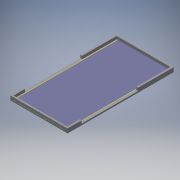
# Autodesk Inventor part: 30_Handyaufnahme
Saved by Autodesk Inventor 2016 (Build 200138000, 138)
## iProperties
Created: 2016-09-16
Part Number: 30_Handyaufnahme
Material: Generisch
Document SubType Name: Modeling
Designer: Bene
Density: 1 g/cm^3
Appearance: Vorgabe
Author: Bene
Autodesk Inventor part; units mm, degrees
(part 1 of 2)
ref_plane "YZ Plane" through (0, 0, 0) normal (1, 0, 0) x (0, 1, 0)
ref_plane "XZ Plane" through (0, 0, 0) normal (0, 1, 0) x (-1, 0, 0)
ref_plane "XY Plane" through (0, 0, 0) normal (0, 0, 1) x (1, 0, 0)
ref_plane "Arbeitsebene1" through (0, 0, 0) normal (0, 0, 1) x (1, 0, 0)
sketch "Skizze1" plane through (0, 0, 0) normal (0, 0, 1) x (1, 0, 0)
  line L0 (0, -3) -> (42, -3) projected
  line L1 (0, -61) -> (0, -3) projected
  line L2 (42, -61) -> (0, -61) projected
  line L3 (42, -3) -> (42, -61) projected
  point P0 (0, 0)
ref_plane "Arbeitsebene2" through (43.5, -39.6821, 19.9558) normal (0, 0, -1) x (-1, 0, 0)
sketch "Skizze2" plane through (43.5, -39.6821, 19.9558) normal (0, 0, -1) x (-1, 0, 0)
  spline S0 degree 3 poles (33.0112, -67.16) (33.0231, -67.1461) (33.0345, -67.1317) (33.045, -67.1168) knots 0 0 0 0 1 1 1 1 construction
  line L0 (33.045, -67.1168) -> (33.045, 67.1168) construction
  spline S1 degree 3 poles (33.045, 67.1168) (33.0378, 67.127) (33.0303, 67.1369) (33.0224, 67.1465) (33.0188, 67.1511) (33.015, 67.1555) (33.0113, 67.16) knots 0 0 0 0 0.680527 0.680527 0.680527 1 1 1 1 construction
  line L1 (33.0113, 67.16) -> (-33.0112, 67.16) construction
  spline S2 degree 3 poles (-33.0112, 67.16) (-33.0231, 67.1461) (-33.0345, 67.1317) (-33.045, 67.1168) knots 0 0 0 0 1 1 1 1 construction
  line L2 (-33.045, 67.1168) -> (-33.045, -67.1168) construction
  spline S3 degree 3 poles (-33.045, -67.1168) (-33.0378, -67.127) (-33.0303, -67.1369) (-33.0224, -67.1465) (-33.0188, -67.1511) (-33.015, -67.1555) (-33.0113, -67.16) knots 0 0 0 0 0.680527 0.680527 0.680527 1 1 1 1 construction
  line L3 (-33.0113, -67.16) -> (33.0112, -67.16) construction
  circle A0 centre (20, -51.9963) radius 1.9005 construction
  circle A1 centre (20, -59.8179) radius 3.8131 construction
  line L4 (-6.8399, -3.5028) -> (-6.8399, -3.3752) construction
  line L5 (-8.0242, -3.5028) -> (-6.8399, -3.5028) construction
  line L6 (-8.0242, -3.3752) -> (-8.0242, -3.5028) construction
  line L7 (-7.8023, -3.3745) -> (-8.0242, -3.3752) construction
  spline S4 degree 3 poles (-7.4456, -3.2197) (-7.4554, -3.2338) (-7.4745, -3.2614) (-7.5108, -3.295) (-7.5488, -3.3237) (-7.5917, -3.3439) (-7.638, -3.3581) (-7.6886, -3.3688) (-7.7439, -3.374) (-7.7824, -3.3743) (-7.8023, -3.3745) knots 0 0 0 0 0.125872 0.246008 0.361529 0.474729 0.592378 0.717307 0.853877 1 1 1 1 construction
  line L8 (-6.2942, -1.4127) -> (-7.4456, -3.2197) construction
  line L9 (-6.2936, -0.4264) -> (-6.2942, -1.4127) construction
  spline S5 degree 3 poles (-6.5588, -0.1303) (-6.5345, -0.1322) (-6.4894, -0.1356) (-6.4278, -0.1541) (-6.3782, -0.1841) (-6.344, -0.2264) (-6.3204, -0.2731) (-6.3032, -0.3223) (-6.2942, -0.3738) (-6.2938, -0.4088) (-6.2936, -0.4264) knots 0 0 0 0 0.16126 0.299397 0.422694 0.539052 0.654895 0.768299 0.88344 1 1 1 1 construction
  line L10 (-6.8508, -0.1303) -> (-6.5588, -0.1303) construction
  line L11 (-6.8508, -0.0028) -> (-6.8508, -0.1303) construction
  line L12 (-5.5009, -0.0028) -> (-6.8508, -0.0028) construction
  line L13 (-5.5009, -0.1303) -> (-5.5009, -0.0028) construction
  line L14 (-5.7867, -0.1303) -> (-5.5009, -0.1303) construction
  spline S6 degree 3 poles (-6.0406, -0.4267) (-6.0397, -0.405) (-6.0379, -0.3639) (-6.0275, -0.3052) (-6.007, -0.2542) (-5.98, -0.2099) (-5.9439, -0.1741) (-5.8986, -0.1488) (-5.8453, -0.1333) (-5.8069, -0.1314) (-5.7867, -0.1303) knots 0 0 0 0 0.146323 0.278524 0.401374 0.515931 0.627633 0.741117 0.863359 1 1 1 1 construction
  line L15 (-6.0406, -1.3884) -> (-6.0406, -0.4267) construction
  line L16 (-4.918, -3.161) -> (-6.0406, -1.3884) construction
  spline S7 degree 3 poles (-4.535, -3.3752) (-4.5587, -3.374) (-4.6039, -3.3717) (-4.6681, -3.362) (-4.7245, -3.344) (-4.7731, -3.3185) (-4.8158, -3.2871) (-4.8537, -3.2502) (-4.8882, -3.208) (-4.9079, -3.1769) (-4.918, -3.161) knots 0 0 0 0 0.153768 0.293392 0.419393 0.535968 0.647417 0.761826 0.877861 1 1 1 1 construction
  line L17 (-4.3245, -3.3752) -> (-4.535, -3.3752) construction
  line L18 (-4.3245, -3.5028) -> (-4.3245, -3.3752) construction
  line L19 (-5.6898, -3.5028) -> (-4.3245, -3.5028) construction
  line L20 (-5.6898, -3.3752) -> (-5.6898, -3.5028) construction
  line L21 (-5.3548, -3.3745) -> (-5.6898, -3.3752) construction
  spline S8 degree 3 poles (-5.1551, -3.2969) (-5.1567, -3.3057) (-5.1597, -3.3228) (-5.1771, -3.3435) (-5.2009, -3.3587) (-5.2422, -3.3674) (-5.2937, -3.3754) (-5.3353, -3.3748) (-5.3548, -3.3745) knots 0 0 0 0 0.113211 0.218392 0.333929 0.468642 0.751865 1 1 1 1 construction
  spline S9 degree 3 poles (-5.2257, -3.1614) (-5.2152, -3.1742) (-5.1958, -3.1977) (-5.1744, -3.2339) (-5.1598, -3.2663) (-5.1566, -3.2873) (-5.1551, -3.2969) knots 0 0 0 0 0.319442 0.590352 0.813067 1 1 1 1 construction
  line L22 (-6.2146, -1.5827) -> (-5.2257, -3.1614) construction
  line L23 (-7.2559, -3.2192) -> (-6.2146, -1.5827) construction
  spline S10 degree 3 poles (-7.283, -3.3017) (-7.2809, -3.2898) (-7.2757, -3.2611) (-7.2632, -3.2346) (-7.2559, -3.2192) knots 0 0 0 0 0.415019 1 1 1 1 construction
  spline S11 degree 3 poles (-7.1806, -3.3752) (-7.1943, -3.3741) (-7.219, -3.372) (-7.2524, -3.359) (-7.2756, -3.334) (-7.2804, -3.3128) (-7.283, -3.3017) knots 0 0 0 0 0.295689 0.535244 0.758161 1 1 1 1 construction
  line L24 (-6.8399, -3.3752) -> (-7.1806, -3.3752) construction
  spline S12 degree 3 poles (-3.5022, -3.1566) (-3.5031, -3.1731) (-3.5048, -3.205) (-3.519, -3.2499) (-3.5424, -3.2883) (-3.5742, -3.3199) (-3.6132, -3.344) (-3.6573, -3.3625) (-3.7074, -3.3727) (-3.7425, -3.3739) (-3.7608, -3.3745) knots 0 0 0 0 0.130398 0.250624 0.365732 0.481486 0.600063 0.724028 0.85602 1 1 1 1 construction
  line L25 (-3.5022, -0.0028) -> (-3.5022, -3.1566) construction
  line L26 (-3.3463, -0.0028) -> (-3.5022, -0.0028) construction
  line L27 (-3.0592, -0.4024) -> (-3.3463, -0.0028) construction
  line L28 (-0.9728, -3.2294) -> (-3.0592, -0.4024) construction
  line L29 (-0.9728, -0.441) -> (-0.9728, -3.2294) construction
  spline S13 degree 3 poles (-1.2708, -0.1303) (-1.2481, -0.1313) (-1.205, -0.1332) (-1.1444, -0.1496) (-1.0921, -0.1758) (-1.0489, -0.2131) (-1.014, -0.2586) (-0.9913, -0.3135) (-0.9749, -0.3746) (-0.9736, -0.4182) (-0.9728, -0.441) knots 0 0 0 0 0.139526 0.264775 0.383096 0.497107 0.612888 0.732612 0.860253 1 1 1 1 construction
  line L30 (-1.4768, -0.1303) -> (-1.2708, -0.1303) construction
  line L31 (-1.4768, -0.0028) -> (-1.4768, -0.1303) construction
  line L32 (-0.2882, -0.0028) -> (-1.4768, -0.0028) construction
  line L33 (-0.2882, -0.1303) -> (-0.2882, -0.0028) construction
  line L34 (-0.5201, -0.1303) -> (-0.2882, -0.1303) construction
  spline S14 degree 3 poles (-0.8009, -0.4412) (-0.7987, -0.4165) (-0.7944, -0.3696) (-0.7729, -0.3049) (-0.7416, -0.2496) (-0.6986, -0.2065) (-0.6522, -0.1738) (-0.6072, -0.1485) (-0.5631, -0.1336) (-0.5341, -0.1314) (-0.5201, -0.1303) knots 0 0 0 0 0.161786 0.306268 0.440748 0.572979 0.699363 0.810681 0.908913 1 1 1 1 construction
  line L35 (-0.8009, -3.1464) -> (-0.8009, -0.4412) construction
  spline S15 degree 3 poles (-0.5473, -3.3752) (-0.559, -3.375) (-0.5837, -3.3746) (-0.6221, -3.3685) (-0.6624, -3.3541) (-0.705, -3.337) (-0.7459, -3.3091) (-0.7757, -3.2652) (-0.795, -3.2098) (-0.7988, -3.1685) (-0.8009, -3.1464) knots 0 0 0 0 0.091352 0.191475 0.301121 0.422609 0.548749 0.678857 0.82774 1 1 1 1 construction
  line L36 (-0.2882, -3.3752) -> (-0.5473, -3.3752) construction
  line L37 (-0.2882, -3.5028) -> (-0.2882, -3.3752) construction
  line L38 (-1.0811, -3.5028) -> (-0.2882, -3.5028) construction
  line L39 (-3.3302, -0.4752) -> (-1.0811, -3.5028) construction
  line L40 (-3.3302, -3.1561) -> (-3.3302, -0.4752) construction
  spline S16 degree 3 poles (-3.0592, -3.3752) (-3.0768, -3.3747) (-3.1108, -3.3737) (-3.1602, -3.3656) (-3.2056, -3.3499) (-3.2475, -3.3292) (-3.2835, -3.2996) (-3.31, -3.2597) (-3.3257, -3.2106) (-3.3286, -3.1749) (-3.3302, -3.1561) knots 0 0 0 0 0.133425 0.258235 0.378828 0.497512 0.612266 0.728756 0.856573 1 1 1 1 construction
  line L41 (-2.8208, -3.3752) -> (-3.0592, -3.3752) construction
  line L42 (-2.8208, -3.5028) -> (-2.8208, -3.3752) construction
  line L43 (-4.0148, -3.5028) -> (-2.8208, -3.5028) construction
  line L44 (-4.0148, -3.3752) -> (-4.0148, -3.5028) construction
  line L45 (-3.7608, -3.3745) -> (-4.0148, -3.3752) construction
  line L46 (-7.4524, 47.564) -> (-6.685, 47.564) construction
  line L47 (-8.7169, 51.0791) -> (-7.4524, 47.564) construction
  line L48 (-8.0576, 51.0791) -> (-8.7169, 51.0791) construction
  line L49 (-7.6848, 50.0505) -> (-8.0576, 51.0791) construction
  line L50 (-6.4202, 50.0505) -> (-7.6848, 50.0505) construction
  line L51 (-6.0636, 51.0791) -> (-6.4202, 50.0505) construction
  line L52 (-5.4206, 51.0791) -> (-6.0636, 51.0791) construction
  line L53 (-6.685, 47.564) -> (-5.4206, 51.0791) construction
  line L54 (-4.2355, 51.0663) -> (-4.8651, 51.0663) construction
  line L55 (-4.2355, 47.5663) -> (-4.2355, 51.0663) construction
  line L56 (-4.8651, 47.5663) -> (-4.2355, 47.5663) construction
  line L57 (-4.8651, 51.0663) -> (-4.8651, 47.5663) construction
  line L58 (4.4914, 49.7461) -> (4.4911, 49.7461) construction
  line L59 (4.4911, 51.0604) -> (4.4911, 49.7461) construction
  line L60 (5.1173, 51.0604) -> (4.4911, 51.0604) construction
  line L61 (5.1177, 47.6325) -> (5.1173, 51.0604) construction
  spline S17 degree 3 poles (4.1058, 47.5637) (4.1579, 47.5645) (4.2591, 47.566) (4.4066, 47.5698) (4.5455, 47.5757) (4.676, 47.5838) (4.7984, 47.5928) (4.9124, 47.6039) (5.018, 47.6171) (5.0853, 47.6275) (5.1177, 47.6325) knots 0 0 0 0 0.153776 0.299112 0.436052 0.564635 0.685507 0.798759 0.903163 1 1 1 1 construction
  spline S18 degree 3 poles (2.9597, 47.8428) (2.9927, 47.8202) (3.0604, 47.7738) (3.1743, 47.7175) (3.2997, 47.6694) (3.4373, 47.6297) (3.5873, 47.5995) (3.7496, 47.5793) (3.9237, 47.5654) (4.0438, 47.5643) (4.1058, 47.5637) knots 0 0 0 0 0.100077 0.205184 0.316963 0.435866 0.563106 0.699421 0.844937 1 1 1 1 construction
  spline S19 degree 3 poles (2.5847, 48.5888) (2.5862, 48.55) (2.5893, 48.474) (2.6081, 48.3629) (2.6392, 48.258) (2.6824, 48.1595) (2.7369, 48.0683) (2.8007, 47.984) (2.8751, 47.908) (2.9313, 47.8647) (2.9597, 47.8428) knots 0 0 0 0 0.134405 0.262714 0.388354 0.511556 0.633904 0.754637 0.876442 1 1 1 1 construction
  spline S20 degree 3 poles (4.1382, 49.7125) (4.0897, 49.7125) (3.9939, 49.7125) (3.8519, 49.7012) (3.7137, 49.6833) (3.5795, 49.6557) (3.449, 49.6206) (3.3219, 49.578) (3.199, 49.5259) (3.0807, 49.4666) (2.9695, 49.3986) (2.8724, 49.3163) (2.7883, 49.2235) (2.7192, 49.1185) (2.664, 49.002) (2.6224, 48.8745) (2.5952, 48.7354) (2.5882, 48.6388) (2.5847, 48.5888) knots 0 0 0 0 0.067532 0.133398 0.198121 0.261385 0.324001 0.386218 0.447841 0.509748 0.570295 0.628891 0.686268 0.74407 0.803241 0.865264 0.930334 1 1 1 1 construction
  spline S21 degree 3 poles (4.2556, 49.7112) (4.2484, 49.7115) (4.2093, 49.7126) (4.1702, 49.7125) (4.1382, 49.7125) knots 0 0 0 0 0.18275 1 1 1 1 construction
  line L62 (4.2556, 49.7112) -> (4.2556, 49.3014) construction
  spline S22 degree 3 poles (4.1382, 49.3018) (4.1728, 49.3022) (4.212, 49.3026) (4.2511, 49.3016) (4.2556, 49.3014) knots 0 0 0 0 0.884897 1 1 1 1 construction
  spline S23 degree 3 poles (3.2143, 48.6113) (3.2153, 48.6385) (3.2172, 48.6913) (3.2291, 48.7679) (3.2493, 48.8395) (3.2762, 48.9065) (3.3108, 48.9685) (3.353, 49.0254) (3.4031, 49.0771) (3.4601, 49.1241) (3.5239, 49.1657) (3.5937, 49.2025) (3.67, 49.2324) (3.752, 49.2577) (3.84, 49.2775) (3.9342, 49.291) (4.0342, 49.2998) (4.1029, 49.3011) (4.1382, 49.3018) knots 0 0 0 0 0.06256 0.121668 0.178098 0.23345 0.287556 0.341282 0.39623 0.45286 0.511168 0.571359 0.634254 0.699626 0.76886 0.841752 0.918713 1 1 1 1 construction
  spline S24 degree 3 poles (4.0675, 47.9797) (4.0361, 47.9802) (3.9752, 47.9813) (3.8859, 47.9885) (3.8016, 48.0011) (3.7218, 48.0179) (3.6473, 48.0409) (3.577, 48.0674) (3.512, 48.1003) (3.4517, 48.137) (3.397, 48.1787) (3.3489, 48.2258) (3.3086, 48.2784) (3.2748, 48.3352) (3.2492, 48.3975) (3.2299, 48.4645) (3.218, 48.5364) (3.2156, 48.5859) (3.2143, 48.6113) knots 0 0 0 0 0.078508 0.152812 0.224327 0.292184 0.35687 0.41968 0.480233 0.539284 0.596432 0.652316 0.707476 0.761976 0.817709 0.875782 0.936291 1 1 1 1 construction
  spline S25 degree 3 poles (4.4911, 48.011) (4.4798, 48.0091) (4.4552, 48.0052) (4.4157, 47.9988) (4.3706, 47.9949) (4.3204, 47.9896) (4.2648, 47.9871) (4.2037, 47.9831) (4.1373, 47.9817) (4.0913, 47.9804) (4.0675, 47.9797) knots 0 0 0 0 0.081247 0.175609 0.281928 0.400632 0.531508 0.674808 0.831962 1 1 1 1 construction
  line L63 (4.4914, 49.2753) -> (4.4911, 48.011) construction
  line L64 (4.4914, 49.2753) -> (4.4914, 49.7461) construction
  line L65 (1.1321, 49.4618) -> (1.1321, 49.0439) construction
  line L66 (-0.1445, 49.0439) -> (1.1321, 49.0439) construction
  line L67 (-0.1445, 49.4618) -> (-0.1445, 49.0439) construction
  line L68 (1.1321, 49.4618) -> (-0.1445, 49.4618) construction
  line L69 (1.3148, 48.0227) -> (-0.2317, 48.0227) construction
  line L70 (1.3148, 50.6523) -> (1.3148, 48.0227) construction
  line L71 (-0.3242, 50.6523) -> (1.3148, 50.6523) construction
  line L72 (-0.3242, 51.0703) -> (-0.3242, 50.6523) construction
  line L73 (1.9444, 51.0703) -> (-0.3242, 51.0703) construction
  line L74 (1.9444, 47.6047) -> (1.9444, 51.0703) construction
  line L75 (-0.2317, 47.6047) -> (1.9444, 47.6047) construction
  line L76 (-0.2317, 48.0227) -> (-0.2317, 47.6047) construction
  line L77 (12.0011, -59.9793) -> (13.1916, -59.9793) construction
  line L78 (12.0016, -58.7456) -> (12.0011, -59.9793) construction
  spline S26 degree 3 poles (13.0636, -58.6238) (13.008, -58.6247) (12.8994, -58.6265) (12.7403, -58.6348) (12.5887, -58.6465) (12.4674, -58.6614) (12.3752, -58.6739) (12.3107, -58.684) (12.25, -58.6938) (12.193, -58.7037) (12.1398, -58.7141) (12.0903, -58.7244) (12.0446, -58.7348) (12.0156, -58.7421) (12.0016, -58.7456) knots 0 0 0 0 0.1557 0.304053 0.446066 0.581493 0.646038 0.70672 0.764353 0.818072 0.868837 0.916143 0.959573 1 1 1 1 construction
  spline S27 degree 3 poles (14.8994, -59.8671) (14.9015, -59.8386) (14.9058, -59.7804) (14.896, -59.691) (14.8756, -59.5986) (14.8423, -59.5034) (14.7975, -59.4054) (14.7407, -59.3045) (14.6723, -59.2006) (14.6072, -59.1128) (14.5468, -59.0432) (14.4936, -58.9936) (14.4336, -58.9473) (14.3673, -58.9037) (14.2943, -58.8638) (14.215, -58.8263) (14.1292, -58.7919) (14.0364, -58.7615) (13.9375, -58.7331) (13.8319, -58.7081) (13.7198, -58.6866) (13.6013, -58.6678) (13.4762, -58.6516) (13.3445, -58.639) (13.2062, -58.6296) (13.1118, -58.6257) (13.0636, -58.6238) knots 0 0 0 0 0.03432 0.070095 0.107736 0.147992 0.191058 0.237276 0.287084 0.340654 0.368703 0.397784 0.428021 0.459755 0.493076 0.528071 0.565217 0.604154 0.645525 0.688944 0.734677 0.782823 0.833245 0.886343 0.941974 1 1 1 1 construction
  spline S28 degree 3 poles (12.97, -61.1861) (13.0055, -61.1857) (13.0754, -61.1849) (13.1791, -61.1799) (13.2802, -61.173) (13.3788, -61.163) (13.4748, -61.1509) (13.5681, -61.1357) (13.6586, -61.1177) (13.7468, -61.0975) (13.8322, -61.0745) (13.915, -61.0482) (13.9954, -61.0202) (14.0729, -60.9887) (14.1481, -60.9554) (14.2206, -60.9189) (14.2904, -60.8797) (14.3574, -60.8382) (14.4214, -60.7945) (14.481, -60.7477) (14.5374, -60.6994) (14.5891, -60.6482) (14.6377, -60.5956) (14.6809, -60.5398) (14.7215, -60.4828) (14.7574, -60.4231) (14.789, -60.3611) (14.817, -60.2971) (14.8412, -60.2309) (14.861, -60.1623) (14.8765, -60.0916) (14.8882, -60.0187) (14.8966, -59.9437) (14.8984, -59.8928) (14.8994, -59.8671) knots 0 0 0 0 0.04072 0.080388 0.119206 0.157214 0.194247 0.23036 0.265776 0.30032 0.33425 0.367443 0.400064 0.432052 0.463561 0.494554 0.525258 0.555487 0.58515 0.614287 0.642511 0.670405 0.697816 0.724748 0.751504 0.77813 0.804755 0.831413 0.858375 0.88569 0.913305 0.941536 0.97047 1 1 1 1 construction
  spline S29 degree 3 poles (12.1025, -61.0811) (12.1275, -61.0888) (12.1807, -61.1053) (12.2668, -61.1251) (12.3633, -61.1429) (12.4695, -61.1584) (12.5844, -61.1704) (12.7068, -61.1792) (12.8361, -61.1851) (12.9247, -61.1858) (12.97, -61.1861) knots 0 0 0 0 0.089617 0.19034 0.302104 0.425118 0.55728 0.697152 0.844869 1 1 1 1 construction
  line L79 (12.2284, -60.7657) -> (12.1025, -61.0811) construction
  spline S30 degree 3 poles (12.97, -60.863) (12.9289, -60.8627) (12.85, -60.8621) (12.7364, -60.856) (12.6323, -60.8482) (12.5375, -60.8356) (12.4508, -60.8206) (12.3708, -60.805) (12.2972, -60.7866) (12.2507, -60.7725) (12.2284, -60.7657) knots 0 0 0 0 0.164208 0.315374 0.454233 0.581106 0.697247 0.80569 0.906846 1 1 1 1 construction
  spline S31 degree 3 poles (14.2999, -59.8832) (14.2981, -59.9225) (14.2946, -59.9992) (14.2748, -60.1101) (14.2447, -60.2138) (14.2029, -60.3098) (14.1501, -60.3984) (14.086, -60.4795) (14.011, -60.5531) (13.9249, -60.618) (13.8303, -60.6754) (13.7282, -60.7257) (13.6189, -60.768) (13.5027, -60.8031) (13.3794, -60.8298) (13.2492, -60.8489) (13.112, -60.8611) (13.0181, -60.8623) (12.97, -60.863) knots 0 0 0 0 0.063442 0.123831 0.181341 0.237349 0.292409 0.347434 0.403696 0.461553 0.521105 0.582039 0.645058 0.710115 0.777776 0.848453 0.922443 1 1 1 1 construction
  spline S32 degree 3 poles (13.0442, -58.9209) (13.0901, -58.9217) (13.1796, -58.9234) (13.3102, -58.9354) (13.434, -58.9546) (13.5509, -58.9814) (13.6609, -59.0158) (13.764, -59.0579) (13.8602, -59.1076) (13.9493, -59.1646) (14.0298, -59.2291) (14.1004, -59.3012) (14.1599, -59.381) (14.2094, -59.4675) (14.2484, -59.5615) (14.2764, -59.6626) (14.2948, -59.7706) (14.2982, -59.845) (14.2999, -59.8832) knots 0 0 0 0 0.077186 0.150659 0.220703 0.287908 0.352389 0.41457 0.475162 0.534436 0.592319 0.648565 0.703868 0.759442 0.816014 0.874682 0.935701 1 1 1 1 construction
  spline S33 degree 3 poles (12.5416, -58.9736) (12.5536, -58.9695) (12.5799, -58.9606) (12.624, -58.9513) (12.6754, -58.9429) (12.7343, -58.9352) (12.801, -58.9301) (12.8753, -58.925) (12.9573, -58.9226) (13.0144, -58.9215) (13.0442, -58.9209) knots 0 0 0 0 0.07529 0.164091 0.266069 0.383443 0.515244 0.661769 0.823927 1 1 1 1 construction
  line L80 (12.5416, -59.6822) -> (12.5416, -58.9736) construction
  line L81 (13.1916, -59.6822) -> (12.5416, -59.6822) construction
  line L82 (13.1916, -59.9793) -> (13.1916, -59.6822) construction
  line L83 (14.6059, -57.957) -> (14.5472, -58.0596) construction
  line L84 (14.5472, -58.0596) -> (14.3623, -58.0596) construction
  line L85 (14.3623, -58.0596) -> (14.3623, -57.0596) construction
  line L86 (14.3623, -57.0596) -> (14.4521, -57.0596) construction
  line L87 (14.4521, -57.0596) -> (14.4521, -57.957) construction
  line L88 (14.4521, -57.957) -> (14.6059, -57.957) construction
  spline S34 degree 3 poles (13.028, -57.9827) (13.0358, -57.9825) (13.0512, -57.9821) (13.0737, -57.9792) (13.0953, -57.9747) (13.1157, -57.9677) (13.1353, -57.9594) (13.1536, -57.9488) (13.1712, -57.9366) (13.1876, -57.9224) (13.2025, -57.9063) (13.2161, -57.8889) (13.2277, -57.8697) (13.2379, -57.8492) (13.2457, -57.8269) (13.2524, -57.8033) (13.2572, -57.7781) (13.2589, -57.7608) (13.2598, -57.7519) knots 0 0 0 0 0.064442 0.126553 0.186779 0.245944 0.30411 0.361785 0.420255 0.479943 0.540286 0.600712 0.661962 0.724472 0.788881 0.856306 0.926348 1 1 1 1 construction
  line L89 (13.2598, -57.7519) -> (13.3495, -57.7519) construction
  spline S35 degree 3 poles (13.3495, -57.7519) (13.3489, -57.7638) (13.3478, -57.7872) (13.3424, -57.8213) (13.3347, -57.8539) (13.3238, -57.8847) (13.3104, -57.9141) (13.2939, -57.9417) (13.2747, -57.9677) (13.2529, -57.9918) (13.2293, -58.0137) (13.204, -58.0329) (13.1772, -58.0489) (13.1491, -58.0624) (13.1196, -58.0725) (13.0887, -58.08) (13.0565, -58.0845) (13.0346, -58.085) (13.0234, -58.0852) knots 0 0 0 0 0.068799 0.135118 0.199001 0.261934 0.323531 0.385435 0.447216 0.510018 0.572511 0.633364 0.693217 0.752555 0.812558 0.873261 0.935543 1 1 1 1 construction
  spline S36 degree 3 poles (13.0234, -58.0852) (13.0124, -58.085) (12.9909, -58.0845) (12.9595, -58.0801) (12.9295, -58.0734) (12.9012, -58.0635) (12.8745, -58.0511) (12.8496, -58.0356) (12.8259, -58.0179) (12.8046, -57.9969) (12.785, -57.9746) (12.7681, -57.9507) (12.7536, -57.9261) (12.7417, -57.9004) (12.7327, -57.8736) (12.726, -57.846) (12.7222, -57.8173) (12.7216, -57.7978) (12.7213, -57.7879) knots 0 0 0 0 0.06948 0.136525 0.200801 0.263983 0.325711 0.387271 0.449493 0.512955 0.576266 0.637575 0.697901 0.757558 0.816588 0.876646 0.937286 1 1 1 1 construction
  spline S37 degree 3 poles (12.7213, -57.7879) (12.7218, -57.774) (12.7228, -57.7464) (12.731, -57.7058) (12.7438, -57.6665) (12.7592, -57.6349) (12.7748, -57.6094) (12.7888, -57.5884) (12.8053, -57.5658) (12.8241, -57.5415) (12.8456, -57.5158) (12.8693, -57.4882) (12.8956, -57.4592) (12.9141, -57.4394) (12.9236, -57.4292) knots 0 0 0 0 0.098701 0.195671 0.29242 0.391339 0.444459 0.504225 0.570348 0.642914 0.72229 0.807923 0.90047 1 1 1 1 construction
  line L90 (12.9236, -57.4292) -> (13.1738, -57.1621) construction
  line L91 (13.1738, -57.1621) -> (12.7085, -57.1621) construction
  line L92 (12.7085, -57.1621) -> (12.7085, -57.0596) construction
  line L93 (12.7085, -57.0596) -> (13.388, -57.0596) construction
  line L94 (13.388, -57.0596) -> (13.0002, -57.4734) construction
  spline S38 degree 3 poles (13.0002, -57.4734) (12.9907, -57.4833) (12.9726, -57.5022) (12.9469, -57.5299) (12.9239, -57.5555) (12.9034, -57.5792) (12.8854, -57.6009) (12.87, -57.6206) (12.8572, -57.6384) (12.8436, -57.6592) (12.8306, -57.6846) (12.8192, -57.7156) (12.8123, -57.7475) (12.8115, -57.7691) (12.8111, -57.7799) knots 0 0 0 0 0.110794 0.212813 0.306078 0.390617 0.467233 0.534451 0.593867 0.644833 0.736221 0.825037 0.911992 1 1 1 1 construction
  spline S39 degree 3 poles (12.8111, -57.7799) (12.8112, -57.7868) (12.8116, -57.8002) (12.8148, -57.8199) (12.8195, -57.839) (12.8267, -57.8572) (12.8353, -57.8749) (12.8464, -57.8916) (12.8591, -57.9078) (12.8738, -57.923) (12.8899, -57.9369) (12.9069, -57.9492) (12.9249, -57.9595) (12.9438, -57.968) (12.9636, -57.9746) (12.9843, -57.9792) (13.0058, -57.9821) (13.0205, -57.9825) (13.028, -57.9827) knots 0 0 0 0 0.061969 0.122129 0.180999 0.240162 0.299865 0.359951 0.421742 0.486546 0.551508 0.614995 0.67724 0.739715 0.803039 0.866487 0.931969 1 1 1 1 construction
  spline S40 degree 3 poles (11.8968, -57.9827) (11.9082, -57.9823) (11.9304, -57.9815) (11.9625, -57.9747) (11.9923, -57.9639) (12.0149, -57.9508) (12.0317, -57.938) (12.0439, -57.927) (12.0557, -57.9145) (12.0666, -57.9002) (12.0772, -57.8845) (12.0875, -57.8675) (12.0971, -57.8487) (12.1029, -57.8356) (12.1059, -57.8288) knots 0 0 0 0 0.122728 0.239717 0.351862 0.463202 0.520261 0.579432 0.640596 0.705298 0.773236 0.844649 0.920046 1 1 1 1 construction
  line L95 (12.1059, -57.8288) -> (12.1957, -57.8288) construction
  spline S41 degree 3 poles (12.1957, -57.8288) (12.1932, -57.8389) (12.1885, -57.8586) (12.1786, -57.8867) (12.1678, -57.9133) (12.1548, -57.9379) (12.1407, -57.961) (12.1245, -57.982) (12.1069, -58.0016) (12.0876, -58.0189) (12.0672, -58.0346) (12.0457, -58.048) (12.0233, -58.0595) (12, -58.069) (11.9757, -58.0762) (11.9506, -58.0814) (11.9246, -58.0847) (11.907, -58.085) (11.898, -58.0852) knots 0 0 0 0 0.072625 0.141977 0.208985 0.273957 0.336889 0.398745 0.460116 0.520825 0.580994 0.640152 0.698622 0.757271 0.816427 0.876254 0.937165 1 1 1 1 construction
  spline S42 degree 3 poles (11.898, -58.0852) (11.885, -58.0848) (11.8591, -58.084) (11.8212, -58.0769) (11.7846, -58.0657) (11.7498, -58.0501) (11.7174, -58.0309) (11.6887, -58.0081) (11.6638, -57.982) (11.643, -57.9532) (11.6267, -57.9225) (11.6147, -57.8908) (11.6074, -57.8583) (11.6064, -57.8364) (11.6059, -57.8254) knots 0 0 0 0 0.090254 0.17854 0.266093 0.354631 0.441886 0.525747 0.608114 0.690197 0.770821 0.848326 0.924012 1 1 1 1 construction
  spline S43 degree 3 poles (11.6059, -57.8254) (11.6063, -57.8148) (11.6069, -57.7941) (11.6124, -57.7639) (11.6217, -57.7355) (11.6346, -57.7086) (11.6513, -57.6835) (11.6715, -57.6602) (11.6953, -57.6385) (11.7134, -57.6261) (11.7227, -57.6197) knots 0 0 0 0 0.128068 0.250608 0.37063 0.490072 0.610375 0.734313 0.863217 1 1 1 1 construction
  spline S44 degree 3 poles (11.7227, -57.6197) (11.7121, -57.6146) (11.6909, -57.6044) (11.6624, -57.5842) (11.6361, -57.5614) (11.6216, -57.5434) (11.6143, -57.5343) knots 0 0 0 0 0.253916 0.503896 0.750255 1 1 1 1 construction
  spline S45 degree 3 poles (11.6143, -57.5343) (11.6095, -57.5277) (11.6, -57.5147) (11.5882, -57.4937) (11.5774, -57.4725) (11.5695, -57.4503) (11.5627, -57.4278) (11.5582, -57.4046) (11.5553, -57.3808) (11.5549, -57.3647) (11.5547, -57.3567) knots 0 0 0 0 0.128146 0.254193 0.378141 0.501381 0.623957 0.747076 0.872865 1 1 1 1 construction
  spline S46 degree 3 poles (11.5547, -57.3567) (11.5552, -57.3426) (11.5562, -57.3147) (11.5653, -57.2734) (11.5796, -57.2331) (11.5994, -57.1944) (11.6241, -57.1583) (11.6532, -57.1259) (11.6869, -57.0983) (11.7242, -57.0751) (11.7648, -57.0566) (11.808, -57.0433) (11.8536, -57.0354) (11.8847, -57.0344) (11.9006, -57.0339) knots 0 0 0 0 0.079635 0.158895 0.23958 0.322382 0.405793 0.487884 0.569711 0.653048 0.737434 0.822573 0.909763 1 1 1 1 construction
  spline S47 degree 3 poles (11.9006, -57.0339) (11.9113, -57.0342) (11.9323, -57.0347) (11.9633, -57.038) (11.9927, -57.0442) (12.021, -57.052) (12.0477, -57.0628) (12.0731, -57.0756) (12.0973, -57.0909) (12.1199, -57.1086) (12.141, -57.1284) (12.1601, -57.1506) (12.1774, -57.1749) (12.1927, -57.2014) (12.2061, -57.2301) (12.2174, -57.261) (12.2272, -57.294) (12.2318, -57.317) (12.2341, -57.3288) knots 0 0 0 0 0.065538 0.128956 0.190367 0.249965 0.308569 0.366415 0.424556 0.483181 0.542251 0.601744 0.662508 0.7245 0.789139 0.856354 0.926299 1 1 1 1 construction
  line L96 (12.2341, -57.3288) -> (12.1444, -57.3288) construction
  spline S48 degree 3 poles (12.1444, -57.3288) (12.1421, -57.3211) (12.1375, -57.3061) (12.1298, -57.2846) (12.121, -57.2648) (12.1115, -57.2467) (12.1016, -57.2301) (12.0904, -57.2153) (12.079, -57.2019) (12.0703, -57.1943) (12.0661, -57.1906) knots 0 0 0 0 0.14977 0.291316 0.425966 0.55216 0.671527 0.786122 0.895325 1 1 1 1 construction
  spline S49 degree 3 poles (12.0661, -57.1906) (12.0605, -57.1863) (12.0493, -57.1777) (12.0311, -57.1666) (12.0119, -57.1572) (11.9915, -57.1495) (11.9699, -57.1438) (11.9473, -57.1396) (11.9235, -57.1369) (11.9073, -57.1366) (11.899, -57.1365) knots 0 0 0 0 0.11826 0.236156 0.35563 0.476249 0.600164 0.728633 0.861326 1 1 1 1 construction
  spline S50 degree 3 poles (11.899, -57.1365) (11.8896, -57.1367) (11.8713, -57.137) (11.8446, -57.1402) (11.8192, -57.1448) (11.7954, -57.152) (11.7727, -57.1606) (11.7518, -57.1719) (11.7321, -57.1846) (11.714, -57.1994) (11.6977, -57.2155) (11.6836, -57.2325) (11.6714, -57.2499) (11.6616, -57.2682) (11.6538, -57.2872) (11.6485, -57.307) (11.6448, -57.3273) (11.6445, -57.3411) (11.6444, -57.348) knots 0 0 0 0 0.076062 0.148732 0.218375 0.285723 0.351058 0.414935 0.478486 0.542169 0.60475 0.664119 0.7215 0.777616 0.832666 0.887858 0.943468 1 1 1 1 construction
  spline S51 degree 3 poles (11.6444, -57.348) (11.6448, -57.3574) (11.6457, -57.3759) (11.6524, -57.4033) (11.6634, -57.4297) (11.6785, -57.4547) (11.6974, -57.4776) (11.7191, -57.4982) (11.7441, -57.5152) (11.7673, -57.527) (11.7878, -57.5349) (11.8054, -57.5404) (11.8251, -57.5448) (11.8466, -57.549) (11.8702, -57.5526) (11.8957, -57.5556) (11.9232, -57.558) (11.9423, -57.559) (11.9521, -57.5596) knots 0 0 0 0 0.066903 0.133472 0.201015 0.271618 0.342884 0.413833 0.485572 0.559817 0.599915 0.643623 0.691922 0.744713 0.801511 0.862871 0.929335 1 1 1 1 construction
  line L97 (11.9521, -57.5596) -> (11.9521, -57.6621) construction
  spline S52 degree 3 poles (11.9521, -57.6621) (11.9397, -57.6624) (11.9155, -57.6629) (11.88, -57.6674) (11.8462, -57.6747) (11.8146, -57.685) (11.7859, -57.6975) (11.7607, -57.7115) (11.7401, -57.7277) (11.7235, -57.7452) (11.7112, -57.7642) (11.7021, -57.7838) (11.6968, -57.8046) (11.696, -57.8187) (11.6957, -57.8258) knots 0 0 0 0 0.110151 0.215684 0.318037 0.418137 0.511656 0.596672 0.673801 0.744527 0.810701 0.874075 0.936704 1 1 1 1 construction
  spline S53 degree 3 poles (11.6957, -57.8258) (11.6958, -57.831) (11.696, -57.8414) (11.699, -57.8566) (11.7034, -57.8714) (11.7097, -57.8855) (11.7178, -57.8991) (11.7276, -57.9121) (11.7392, -57.9246) (11.7525, -57.9365) (11.7672, -57.9472) (11.7829, -57.9567) (11.7997, -57.9647) (11.8173, -57.9714) (11.8359, -57.9763) (11.8554, -57.9799) (11.8758, -57.9822) (11.8897, -57.9825) (11.8968, -57.9827) knots 0 0 0 0 0.055265 0.109948 0.163898 0.21807 0.273285 0.330884 0.390478 0.454119 0.518941 0.583379 0.648575 0.715078 0.782538 0.852347 0.924941 1 1 1 1 construction
  line L98 (12.4828, -55.9076) -> (12.546, -55.9076) construction
  line L99 (12.546, -55.9076) -> (12.4536, -56.6076) construction
  line L100 (12.4536, -56.6076) -> (12.4446, -56.6076) construction
  line L101 (12.4446, -56.6076) -> (12.1556, -56.0333) construction
  line L102 (12.1556, -56.0333) -> (11.8673, -56.6076) construction
  line L103 (11.8673, -56.6076) -> (11.8582, -56.6076) construction
  line L104 (11.8582, -56.6076) -> (11.7652, -55.9076) construction
  line L105 (11.7652, -55.9076) -> (11.8283, -55.9076) construction
  line L106 (11.8283, -55.9076) -> (11.8954, -56.4113) construction
  line L107 (11.8954, -56.4113) -> (12.148, -55.9076) construction
  line L108 (12.148, -55.9076) -> (12.1622, -55.9076) construction
  line L109 (12.1622, -55.9076) -> (12.4159, -56.4124) construction
  line L110 (12.4159, -56.4124) -> (12.4828, -55.9076) construction
  spline S54 degree 3 poles (13.3178, -55.957) (13.3176, -55.9609) (13.3172, -55.9686) (13.3138, -55.9797) (13.3083, -55.9897) (13.3009, -55.9986) (13.292, -56.006) (13.282, -56.0114) (13.271, -56.0146) (13.2634, -56.0151) (13.2595, -56.0153) knots 0 0 0 0 0.129097 0.252046 0.373905 0.501038 0.628171 0.751376 0.872426 1 1 1 1 construction
  spline S55 degree 3 poles (13.2595, -56.0153) (13.2556, -56.0151) (13.2479, -56.0146) (13.2369, -56.0115) (13.2269, -56.006) (13.218, -55.9986) (13.2106, -55.9897) (13.2049, -55.9797) (13.2018, -55.9686) (13.2014, -55.9609) (13.2011, -55.957) knots 0 0 0 0 0.127519 0.249986 0.371792 0.49887 0.625948 0.748492 0.870959 1 1 1 1 construction
  spline S56 degree 3 poles (13.2011, -55.957) (13.2014, -55.9531) (13.2018, -55.9455) (13.2049, -55.9345) (13.2107, -55.9245) (13.2179, -55.9155) (13.2269, -55.9081) (13.2369, -55.9026) (13.2479, -55.8993) (13.2556, -55.8989) (13.2595, -55.8986) knots 0 0 0 0 0.126178 0.248821 0.37154 0.499984 0.627244 0.749226 0.872298 1 1 1 1 construction
  spline S57 degree 3 poles (13.2595, -55.8986) (13.2634, -55.8988) (13.271, -55.8993) (13.2819, -55.9027) (13.292, -55.908) (13.301, -55.9155) (13.3083, -55.9245) (13.3138, -55.9345) (13.3171, -55.9455) (13.3176, -55.9531) (13.3178, -55.957) knots 0 0 0 0 0.127757 0.249414 0.372796 0.500111 0.62861 0.750643 0.873768 1 1 1 1 construction
  spline S58 degree 3 poles (14.1966, -56.5538) (14.202, -56.5536) (14.2128, -56.5533) (14.2286, -56.5514) (14.2436, -56.548) (14.258, -56.5434) (14.2717, -56.5375) (14.2847, -56.5301) (14.2969, -56.5214) (14.3084, -56.5114) (14.3189, -56.5004) (14.3282, -56.4881) (14.3364, -56.4747) (14.3434, -56.4603) (14.3492, -56.4448) (14.3536, -56.4282) (14.3571, -56.4106) (14.3582, -56.3985) (14.3588, -56.3922) knots 0 0 0 0 0.064439 0.126547 0.186887 0.245878 0.304041 0.362191 0.420976 0.48066 0.5406 0.600689 0.661936 0.724443 0.789038 0.856314 0.926352 1 1 1 1 construction
  line L111 (14.3588, -56.3922) -> (14.4216, -56.3922) construction
  spline S59 degree 3 poles (14.4216, -56.3922) (14.4212, -56.4006) (14.4204, -56.4169) (14.4167, -56.4408) (14.4113, -56.4636) (14.4036, -56.4852) (14.3942, -56.5057) (14.3828, -56.5251) (14.3694, -56.5433) (14.3542, -56.5601) (14.3376, -56.5756) (14.3197, -56.5889) (14.301, -56.6002) (14.2814, -56.6096) (14.2607, -56.6166) (14.2391, -56.6219) (14.2165, -56.625) (14.2012, -56.6254) (14.1933, -56.6256) knots 0 0 0 0 0.068791 0.135103 0.198979 0.261904 0.323495 0.385195 0.446969 0.509765 0.572251 0.633405 0.693251 0.752583 0.812579 0.873275 0.93555 1 1 1 1 construction
  spline S60 degree 3 poles (14.1933, -56.6256) (14.1857, -56.6254) (14.1706, -56.625) (14.1486, -56.622) (14.1276, -56.6172) (14.1078, -56.6106) (14.0892, -56.6016) (14.0717, -56.5909) (14.0551, -56.5784) (14.0402, -56.5638) (14.0265, -56.5481) (14.0147, -56.5314) (14.0045, -56.5142) (13.9961, -56.4963) (13.9899, -56.4775) (13.9852, -56.4581) (13.9825, -56.438) (13.9821, -56.4244) (13.9819, -56.4175) knots 0 0 0 0 0.069475 0.136517 0.200789 0.26383 0.325735 0.387291 0.449509 0.512968 0.576275 0.63758 0.697903 0.757172 0.816599 0.876653 0.93729 1 1 1 1 construction
  spline S61 degree 3 poles (13.9819, -56.4175) (13.9822, -56.4077) (13.9829, -56.3884) (13.9886, -56.36) (13.9976, -56.3325) (14.0084, -56.3103) (14.0193, -56.2925) (14.0291, -56.2778) (14.0406, -56.262) (14.054, -56.2451) (14.0689, -56.227) (14.0855, -56.2077) (14.1039, -56.1874) (14.1168, -56.1735) (14.1235, -56.1663) knots 0 0 0 0 0.098702 0.195672 0.292422 0.391343 0.444462 0.504229 0.570352 0.642546 0.722288 0.807921 0.90047 1 1 1 1 construction
  line L112 (14.1235, -56.1663) -> (14.2987, -55.9794) construction
  line L113 (14.2987, -55.9794) -> (13.9729, -55.9794) construction
  line L114 (13.9729, -55.9794) -> (13.9729, -55.9076) construction
  line L115 (13.9729, -55.9076) -> (14.4486, -55.9076) construction
  line L116 (14.4486, -55.9076) -> (14.1771, -56.1973) construction
  spline S62 degree 3 poles (14.1771, -56.1973) (14.1705, -56.2042) (14.1578, -56.2175) (14.1398, -56.2368) (14.1237, -56.2548) (14.1093, -56.2713) (14.0969, -56.2866) (14.0859, -56.3002) (14.0772, -56.3128) (14.0676, -56.3273) (14.0584, -56.3451) (14.0504, -56.3668) (14.0456, -56.3892) (14.045, -56.4043) (14.0447, -56.4119) knots 0 0 0 0 0.110803 0.212829 0.306101 0.390647 0.466924 0.534481 0.593587 0.644557 0.7362 0.825024 0.911986 1 1 1 1 construction
  spline S63 degree 3 poles (14.0447, -56.4119) (14.0448, -56.4166) (14.0451, -56.426) (14.0473, -56.4398) (14.0506, -56.4532) (14.0554, -56.466) (14.0618, -56.4783) (14.0694, -56.49) (14.0783, -56.5014) (14.0886, -56.512) (14.0999, -56.5217) (14.1118, -56.5304) (14.1244, -56.5376) (14.1377, -56.5435) (14.1515, -56.5481) (14.166, -56.5513) (14.181, -56.5534) (14.1913, -56.5536) (14.1966, -56.5538) knots 0 0 0 0 0.061965 0.122122 0.180988 0.239933 0.299906 0.359989 0.421776 0.486576 0.551535 0.615018 0.677259 0.73973 0.80305 0.866495 0.931973 1 1 1 1 construction
  spline S64 degree 3 poles (13.6761, -55.8897) (13.6816, -55.8898) (13.6925, -55.8899) (13.7086, -55.8918) (13.7243, -55.8949) (13.7395, -55.8992) (13.7545, -55.9044) (13.7689, -55.9113) (13.7829, -55.9191) (13.7966, -55.9281) (13.8096, -55.9383) (13.822, -55.9497) (13.8335, -55.9624) (13.8443, -55.9763) (13.8545, -55.9913) (13.8638, -56.0074) (13.8725, -56.0248) (13.8804, -56.0435) (13.8875, -56.0637) (13.8937, -56.0857) (13.8986, -56.1098) (13.9028, -56.1356) (13.9062, -56.1633) (13.9085, -56.193) (13.9099, -56.2245) (13.91, -56.2462) (13.9101, -56.2573) knots 0 0 0 0 0.033787 0.066622 0.099285 0.131361 0.163585 0.196104 0.228902 0.262158 0.295991 0.330218 0.36506 0.400951 0.43762 0.475708 0.515381 0.556414 0.599765 0.646424 0.696431 0.749782 0.806573 0.867436 0.931887 1 1 1 1 construction
  spline S65 degree 3 poles (13.9101, -56.2573) (13.91, -56.2685) (13.9099, -56.2903) (13.9085, -56.3221) (13.9061, -56.3519) (13.9029, -56.3797) (13.899, -56.4056) (13.8937, -56.4294) (13.8878, -56.4514) (13.8809, -56.4715) (13.8731, -56.49) (13.8646, -56.5073) (13.8551, -56.5233) (13.8451, -56.5383) (13.8342, -56.5521) (13.8227, -56.5648) (13.8102, -56.5762) (13.7972, -56.5866) (13.7834, -56.5957) (13.7692, -56.6037) (13.7547, -56.6105) (13.7397, -56.6159) (13.7243, -56.6203) (13.7086, -56.6234) (13.6925, -56.6253) (13.6816, -56.6255) (13.6761, -56.6256) knots 0 0 0 0 0.068595 0.133246 0.194313 0.251279 0.304513 0.354235 0.400481 0.443411 0.484015 0.523252 0.561042 0.5979 0.633518 0.668314 0.702496 0.736685 0.770293 0.803437 0.835913 0.86846 0.900847 0.933467 0.966258 1 1 1 1 construction
  spline S66 degree 3 poles (13.6761, -56.6256) (13.6705, -56.6255) (13.6594, -56.6253) (13.6431, -56.6234) (13.6271, -56.6203) (13.6115, -56.6159) (13.5963, -56.6105) (13.5815, -56.6037) (13.5671, -56.5957) (13.5532, -56.5864) (13.5398, -56.576) (13.5271, -56.5643) (13.5151, -56.5513) (13.5038, -56.5372) (13.4934, -56.5217) (13.4835, -56.5052) (13.4746, -56.4872) (13.4661, -56.4682) (13.4587, -56.4475) (13.452, -56.4254) (13.4466, -56.4015) (13.4422, -56.3759) (13.4387, -56.3486) (13.4362, -56.3197) (13.4348, -56.289) (13.4346, -56.2681) (13.4345, -56.2573) knots 0 0 0 0 0.033788 0.067194 0.099862 0.132567 0.165151 0.197913 0.231319 0.265083 0.299255 0.334399 0.369943 0.406284 0.444064 0.482998 0.523354 0.565537 0.609613 0.656391 0.705885 0.758325 0.813832 0.872795 0.934722 1 1 1 1 construction
  spline S67 degree 3 poles (13.4345, -56.2573) (13.4346, -56.2466) (13.4348, -56.2258) (13.4362, -56.1953) (13.4387, -56.1665) (13.442, -56.1393) (13.4465, -56.1139) (13.452, -56.0901) (13.4581, -56.0679) (13.4657, -56.0475) (13.474, -56.0285) (13.483, -56.0108) (13.4926, -55.9941) (13.5032, -55.9787) (13.5144, -55.9645) (13.5265, -55.9516) (13.5393, -55.9397) (13.5527, -55.9292) (13.5668, -55.92) (13.5812, -55.9117) (13.5962, -55.9051) (13.6113, -55.8994) (13.627, -55.895) (13.643, -55.892) (13.6594, -55.8899) (13.6705, -55.8897) (13.6761, -55.8897) knots 0 0 0 0 0.065063 0.126773 0.185516 0.240765 0.29298 0.34225 0.388919 0.432776 0.474628 0.514775 0.553606 0.591426 0.628028 0.663804 0.698984 0.733591 0.767628 0.801208 0.834264 0.866981 0.89972 0.932702 0.966176 1 1 1 1 construction
  line L117 (13.0665, -56.5358) -> (13.0665, -56.6076) construction
  line L118 (13.0665, -56.6076) -> (12.6357, -56.6076) construction
  line L119 (12.6357, -56.6076) -> (13.0037, -55.8897) construction
  line L120 (13.0037, -55.8897) -> (13.058, -55.9195) construction
  line L121 (13.058, -55.9195) -> (12.742, -56.5358) construction
  line L122 (12.742, -56.5358) -> (13.0665, -56.5358) construction
  line L123 (11.6216, -55.9076) -> (11.6216, -56.6076) construction
  line L124 (11.6216, -56.6076) -> (11.4844, -56.6076) construction
  spline S68 degree 3 poles (11.4844, -56.6076) (11.4749, -56.6076) (11.4568, -56.6076) (11.4309, -56.607) (11.4073, -56.6062) (11.3862, -56.6051) (11.3674, -56.6037) (11.3511, -56.6019) (11.3371, -56.6) (11.3287, -56.598) (11.3249, -56.5971) knots 0 0 0 0 0.176956 0.339055 0.486318 0.618781 0.735619 0.838742 0.926457 1 1 1 1 construction
  spline S69 degree 3 poles (11.3249, -56.5971) (11.3201, -56.5958) (11.3105, -56.5932) (11.2967, -56.5879) (11.2836, -56.5817) (11.2711, -56.5746) (11.2594, -56.5663) (11.2483, -56.5573) (11.2379, -56.5471) (11.2283, -56.536) (11.2194, -56.5242) (11.2118, -56.5115) (11.2054, -56.498) (11.1999, -56.4838) (11.196, -56.4689) (11.193, -56.4532) (11.1911, -56.4368) (11.191, -56.4256) (11.1909, -56.4198) knots 0 0 0 0 0.062481 0.12349 0.183411 0.243153 0.302127 0.36171 0.421842 0.482932 0.544552 0.605681 0.66768 0.729984 0.794551 0.860346 0.928907 1 1 1 1 construction
  spline S70 degree 3 poles (11.1909, -56.4198) (11.1909, -56.4141) (11.1911, -56.4028) (11.1931, -56.3864) (11.1958, -56.3706) (11.1999, -56.3556) (11.2052, -56.3415) (11.2115, -56.328) (11.2191, -56.3154) (11.2279, -56.3036) (11.2376, -56.2926) (11.2482, -56.2825) (11.2598, -56.2734) (11.2722, -56.2652) (11.2856, -56.2581) (11.2997, -56.2518) (11.3148, -56.2464) (11.3252, -56.2436) (11.3305, -56.2422) knots 0 0 0 0 0.070119 0.137192 0.202016 0.264631 0.326117 0.38601 0.445812 0.505298 0.564633 0.624283 0.683902 0.743953 0.805388 0.868388 0.933084 1 1 1 1 construction
  spline S71 degree 3 poles (11.3305, -56.2422) (11.3349, -56.2413) (11.3445, -56.2392) (11.3604, -56.2369) (11.3788, -56.235) (11.3998, -56.2335) (11.4233, -56.2323) (11.4495, -56.2313) (11.4782, -56.2307) (11.4983, -56.2307) (11.5088, -56.2307) knots 0 0 0 0 0.075173 0.164746 0.268017 0.385912 0.517789 0.663691 0.824413 1 1 1 1 construction
  line L125 (11.5088, -56.2307) -> (11.5588, -56.2307) construction
  line L126 (11.5588, -56.2307) -> (11.5588, -55.9076) construction
  line L127 (11.5588, -55.9076) -> (11.6216, -55.9076) construction
  spline S72 degree 3 poles (12.5418, -57.1301) (12.5415, -57.1357) (12.5409, -57.1467) (12.5364, -57.1626) (12.5283, -57.1768) (12.5178, -57.1896) (12.5051, -57.2001) (12.4908, -57.208) (12.475, -57.2124) (12.4641, -57.2131) (12.4585, -57.2134) knots 0 0 0 0 0.129041 0.251508 0.374052 0.50113 0.628208 0.750014 0.872481 1 1 1 1 construction
  spline S73 degree 3 poles (12.4585, -57.2134) (12.4529, -57.2131) (12.4421, -57.2125) (12.4263, -57.2079) (12.412, -57.2002) (12.3992, -57.1895) (12.3887, -57.1769) (12.3809, -57.1625) (12.3761, -57.1467) (12.3755, -57.1357) (12.3752, -57.1301) knots 0 0 0 0 0.127574 0.248624 0.371829 0.498962 0.626095 0.747954 0.870903 1 1 1 1 construction
  spline S74 degree 3 poles (12.3752, -57.1301) (12.3755, -57.1246) (12.3761, -57.1137) (12.3809, -57.0981) (12.3887, -57.0837) (12.3993, -57.0711) (12.4119, -57.0602) (12.4264, -57.0526) (12.442, -57.0476) (12.4529, -57.0471) (12.4585, -57.0468) knots 0 0 0 0 0.126257 0.249407 0.371465 0.498805 0.627129 0.750535 0.872218 1 1 1 1 construction
  spline S75 degree 3 poles (12.4585, -57.0468) (12.4641, -57.0471) (12.475, -57.0477) (12.4907, -57.0525) (12.5051, -57.0603) (12.5177, -57.071) (12.5283, -57.0838) (12.5364, -57.098) (12.5408, -57.1137) (12.5415, -57.1246) (12.5418, -57.1301) knots 0 0 0 0 0.127728 0.250825 0.372831 0.501099 0.628385 0.751129 0.873797 1 1 1 1 construction
  line L128 (13.5595, -58.0852) -> (13.4649, -58.0852) construction
  line L129 (13.4649, -58.0852) -> (13.8832, -56.9185) construction
  line L130 (13.8832, -56.9185) -> (13.9777, -56.9185) construction
  line L131 (13.9777, -56.9185) -> (13.5595, -58.0852) construction
  spline S76 degree 3 poles (7.3705, 48.632) (7.3707, 48.6317) (7.3982, 48.5833) (7.4551, 48.4839) (7.5131, 48.3855) (7.543, 48.3349) knots 0.486442 0.486442 0.486442 0.486442 0.487929 0.736354 1 1 1 1 construction
  line L132 (7.3705, 48.632) -> (7.7845, 49.0123) construction
  line L133 (8.7157, 47.5663) -> (7.7845, 49.0123) construction
  line L134 (8.0043, 47.5663) -> (8.7157, 47.5663) construction
  line L135 (7.543, 48.3349) -> (8.0043, 47.5663) construction
  line L136 (7.6079, 49.2865) -> (7.2062, 48.9161) construction
  line L137 (7.2011, 48.9162) -> (7.2062, 48.9161) construction
  spline S77 degree 3 poles (6.8747, 48.3303) (6.9042, 48.3803) (6.9613, 48.4771) (7.0446, 48.621) (7.124, 48.7663) (7.1748, 48.8652) (7.2011, 48.9162) knots 0 0 0 0 0.259536 0.502892 0.743355 1 1 1 1 construction
  line L138 (6.4186, 47.5663) -> (6.8747, 48.3303) construction
  line L139 (5.7126, 47.5663) -> (6.4186, 47.5663) construction
  line L140 (6.853, 49.2728) -> (5.7126, 47.5663) construction
  line L141 (5.6746, 51.0663) -> (6.853, 49.2728) construction
  line L142 (6.386, 51.0663) -> (5.6746, 51.0663) construction
  line L143 (6.8426, 50.321) -> (6.386, 51.0663) construction
  spline S78 degree 3 poles (7.244, 49.6571) (7.2157, 49.709) (7.1584, 49.814) (7.0814, 49.944) (7.0155, 50.0512) (6.9612, 50.1367) (6.9039, 50.2277) (6.8634, 50.2893) (6.8426, 50.321) knots 0 0 0 0 0.228665 0.46209 0.58414 0.715131 0.853443 1 1 1 1 construction
  line L144 (7.2606, 49.6576) -> (7.244, 49.6571) construction
  spline S79 degree 3 poles (7.6296, 50.3206) (7.6109, 50.2889) (7.5744, 50.2271) (7.5204, 50.1372) (7.4721, 50.0507) (7.4101, 49.9441) (7.339, 49.8141) (7.2865, 49.7094) (7.2606, 49.6576) knots 0 0 0 0 0.145219 0.283914 0.414271 0.536845 0.771226 1 1 1 1 construction
  line L145 (8.0586, 51.0663) -> (7.6296, 50.3206) construction
  line L146 (8.7593, 51.0663) -> (8.0586, 51.0663) construction
  line L147 (7.6079, 49.2865) -> (8.7593, 51.0663) construction
  spline S80 degree 3 poles (-2.7664, 49.3869) (-2.7925, 49.378) (-2.8443, 49.3604) (-2.9192, 49.3292) (-2.9908, 49.2941) (-3.0588, 49.2551) (-3.1234, 49.2127) (-3.1842, 49.1662) (-3.242, 49.1167) (-3.2954, 49.0631) (-3.3446, 49.0065) (-3.3878, 48.9462) (-3.4244, 48.8824) (-3.4542, 48.8151) (-3.4782, 48.7445) (-3.4959, 48.6706) (-3.5075, 48.5934) (-3.5095, 48.5408) (-3.5106, 48.5141) knots 0 0 0 0 0.06741 0.133204 0.19788 0.261695 0.32417 0.386319 0.448071 0.509655 0.570649 0.630769 0.690249 0.749693 0.809876 0.871813 0.934841 1 1 1 1 construction
  line L148 (-2.7659, 49.3964) -> (-2.7664, 49.3869) construction
  spline S81 degree 3 poles (-3.3472, 50.1153) (-3.3349, 50.0707) (-3.3108, 49.9839) (-3.2615, 49.8623) (-3.2047, 49.7521) (-3.1391, 49.6538) (-3.0632, 49.5678) (-2.9755, 49.4954) (-2.8758, 49.4369) (-2.803, 49.4101) (-2.7659, 49.3964) knots 0 0 0 0 0.14327 0.278725 0.40581 0.526858 0.643929 0.759889 0.877735 1 1 1 1 construction
  spline S82 degree 3 poles (-3.6576, 51.066) (-3.6466, 51.046) (-3.6217, 51.0008) (-3.5892, 50.9207) (-3.5536, 50.823) (-3.5167, 50.7078) (-3.4774, 50.5776) (-3.4361, 50.4341) (-3.3913, 50.2789) (-3.3623, 50.1711) (-3.3472, 50.1153) knots 0 0 0 0 0.068313 0.154382 0.258376 0.379867 0.516435 0.665591 0.826896 1 1 1 1 construction
  line L149 (-3.0053, 51.0663) -> (-3.6576, 51.066) construction
  spline S83 degree 3 poles (-2.744, 50.2297) (-2.757, 50.2815) (-2.7818, 50.3809) (-2.8185, 50.5233) (-2.8547, 50.6521) (-2.89, 50.7665) (-2.921, 50.8661) (-2.9525, 50.9479) (-2.9771, 51.0142) (-2.9968, 51.0506) (-3.0053, 51.0663) knots 0 0 0 0 0.182491 0.349827 0.502428 0.639426 0.758995 0.858608 0.93903 1 1 1 1 construction
  spline S84 degree 3 poles (-1.9861, 49.5849) (-2.0126, 49.5851) (-2.0639, 49.5857) (-2.1385, 49.5928) (-2.2085, 49.6026) (-2.274, 49.6187) (-2.3347, 49.6397) (-2.3908, 49.6656) (-2.442, 49.6962) (-2.4892, 49.7315) (-2.5317, 49.7734) (-2.5715, 49.8204) (-2.6079, 49.8736) (-2.6411, 49.9331) (-2.6712, 49.9986) (-2.6991, 50.0701) (-2.7235, 50.1478) (-2.737, 50.2019) (-2.744, 50.2297) knots 0 0 0 0 0.071993 0.139434 0.203729 0.264242 0.322663 0.378208 0.432003 0.484663 0.538106 0.593858 0.652085 0.71331 0.778783 0.848283 0.921881 1 1 1 1 construction
  line L150 (-1.6041, 49.5849) -> (-1.9861, 49.5849) construction
  line L151 (-1.6041, 51.066) -> (-1.6041, 49.5849) construction
  line L152 (-0.9779, 51.066) -> (-1.6041, 51.066) construction
  line L153 (-0.9775, 47.6391) -> (-0.9779, 51.066) construction
  spline S85 degree 3 poles (-1.9914, 47.5657) (-1.8981, 47.567) (-1.7152, 47.5696) (-1.4898, 47.5821) (-1.3181, 47.5978) (-1.1978, 47.6092) (-1.0851, 47.6231) (-1.0125, 47.6339) (-0.9775, 47.6391) knots 0 0 0 0 0.275036 0.539383 0.66533 0.78357 0.895565 1 1 1 1 construction
  spline S86 degree 3 poles (-3.1792, 47.8448) (-3.1454, 47.8212) (-3.076, 47.7729) (-2.9588, 47.7155) (-2.8301, 47.6672) (-2.6887, 47.629) (-2.5343, 47.6005) (-2.366, 47.5793) (-2.1834, 47.5679) (-2.0569, 47.5664) (-1.9914, 47.5657) knots 0 0 0 0 0.099663 0.204095 0.314604 0.431784 0.557677 0.694165 0.841625 1 1 1 1 construction
  spline S87 degree 3 poles (-3.5106, 48.5141) (-3.5093, 48.4799) (-3.5069, 48.4128) (-3.4908, 48.3149) (-3.4642, 48.2224) (-3.4278, 48.1352) (-3.3811, 48.0536) (-3.3235, 47.978) (-3.2566, 47.9071) (-3.2053, 47.8658) (-3.1792, 47.8448) knots 0 0 0 0 0.132402 0.259419 0.382764 0.503923 0.62387 0.745646 0.870503 1 1 1 1 construction
  spline S88 degree 3 poles (1.2055, -33.008) (1.1759, -32.9799) (1.1302, -32.9415) (1.0855, -32.8848) (1.0476, -32.8362) (1.0409, -32.7914) (1.0224, -32.7673) knots 0 0 0 0 0.401359 0.579129 0.708069 1 1 1 1 construction